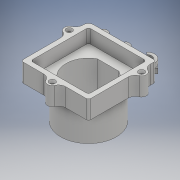
# Autodesk Inventor part: MS_FocusSliderv11
Saved by Autodesk Inventor 2017 (Build 210142000, 142)
## iProperties
Created: 2017-12-13
Part Number: MS_FocusSliderv11
Material: Generic
Document SubType Name: Modeling
Designer: andrew
Density: 1 g/cm^3
Appearance: Default
Author: andrew
Autodesk Inventor part; units mm, degrees
note: some values were not read from the file. Chosen so that the rebuilt part matches the saved one: edges of "Chamfer1".
ref_plane "YZ Plane" through (0, 0, 0) normal (1, 0, 0) x (0, 1, 0)
ref_plane "XZ Plane" through (0, 0, 0) normal (0, 1, 0) x (-1, 0, 0)
sketch "Sketch1" plane through (0, 0, 0) normal (0, 0, 1) x (1, 0, 0)
  circle A0 centre (0, 0) radius 5.75
  line L0 (2.2382, 4.0759) -> (-2.2382, 4.0759)
  arc A1 (-2.2382, 4.0759) -> (2.2382, 4.0759) centre (0, 0) ccw
  dimension "d0" = 11.5
  dimension "d50" = 9.3
  constraints: 2 centre point, 2 end point, 2 point on circle, 1 coincident
  measures "d0" diameter of A0
  measures "d50" diameter of A1
extrude "Extrusion1" add sketch "Sketch1" along normal blind 7
sketch "Sketch2" plane through (0, 0, 0) normal (0, 0, -1) x (-1, 0, 0)
  line L0 (-1.25, 5.125) -> (1.25, 5.125) construction
  circle A0 centre (0, 0) radius 5.75 construction
  line L1 (0, 0) -> (0, 9.5083) construction
  circle A1 centre (0, 0) radius 5.75 construction
  line L2 (0, 5.75) -> (0, 7.7304) construction
  line L3 (0, 5.125) -> (0, 7.5987) construction
  line L4 (-1.25, 5.125) -> (-1.25, 6.125) construction
  line L5 (-1.25, 6.125) -> (1.25, 6.125)
  line L6 (1.25, 6.125) -> (1.25, 4.5986)
  line L7 (1.25, 4.5986) -> (-1.25, 4.5986)
  line L8 (-1.25, 4.5986) -> (-1.25, 6.125)
  dimension "d3" = 2.5
  dimension "d4" = 1
  constraints: 18 end point, 3 vertical, 2 horizontal, 2 parallel, 2 point on line, 1 midpoint, 1 perpendicular, 1 vertical alignment, 1 other
  measures "d3" distance of L0.start L0.end
  measures "d4" distance of L0.start L4.end
extrude "Extrusion2" add sketch "Sketch2" against normal blind 5
sketch "Sketch3" plane through (0, 0, 7) normal (0, 0, 1) x (1, 0, 0)
  line L0 (6.5, 7) -> (-6, 7)
  arc A0 (-6, 7) -> (-7, 6) centre (-6, 6) ccw
  arc A1 (-7, -6.5) -> (-6.5, -7) centre (-6.5, -6.5) ccw
  arc A2 (6.5, -7) -> (7, -6.5) centre (6.5, -6.5) ccw
  arc A3 (7, 6.5) -> (6.5, 7) centre (6.5, 6.5) ccw
  line L1 (-5.5, 6) -> (5.5, 6)
  line L2 (6, 5.5) -> (6, -5.5)
  line L3 (5.5, -6) -> (-5.5, -6)
  line L4 (-6, -5.5) -> (-6, 5.5)
  arc A4 (-5.5, 6) -> (-6, 5.5) centre (-5.5, 5.5) ccw
  arc A5 (6, 5.5) -> (5.5, 6) centre (5.5, 5.5) ccw
  arc A6 (5.5, -6) -> (6, -5.5) centre (5.5, -5.5) ccw
  arc A7 (-6, -5.5) -> (-5.5, -6) centre (-5.5, -5.5) ccw
  line L5 (-10.9736, 8.9739) -> (-4.3472, 8.9739) construction
  arc A8 (-7.9, 4.4165) -> (-7.9, 2.5835) centre (-7.5, 3.5) ccw
  circle A9 centre (-7.5, 3.5) radius 0.375
  arc A10 (-0.9165, -7.9) -> (0.9165, -7.9) centre (0, -7.5) ccw
  circle A11 centre (0, -7.5) radius 0.375
  arc A12 (7.9, 2.5835) -> (7.9, 4.4165) centre (7.5, 3.5) ccw
  circle A13 centre (7.5, 3.5) radius 0.375
  line L6 (-7, 6) -> (-7, 5.7913)
  line L7 (-7, 1.2087) -> (-7, -6.5)
  arc A14 (-7.9, 4.4165) -> (-7, 5.7913) centre (-8.5, 5.7913) ccw
  arc A15 (-7, 1.2087) -> (-7.9, 2.5835) centre (-8.5, 1.2087) ccw
  line L8 (-6.5, -7) -> (-2.2913, -7)
  line L9 (2.2913, -7) -> (6.5, -7)
  arc A16 (-0.9165, -7.9) -> (-2.2913, -7) centre (-2.2913, -8.5) ccw
  arc A17 (2.2913, -7) -> (0.9165, -7.9) centre (2.2913, -8.5) ccw
  line L10 (7, -6.5) -> (7, 1.2087)
  line L11 (7, 5.7913) -> (7, 6.5)
  arc A18 (7, 5.7913) -> (7.9, 4.4165) centre (8.5, 5.7913) ccw
  arc A19 (7.9, 2.5835) -> (7, 1.2087) centre (8.5, 1.2087) ccw
  arc A20 (-2.2382, 4.0759) -> (2.2382, 4.0759) centre (0, 0) ccw
  line L12 (-2.2382, 4.0759) -> (2.2382, 4.0759) projected
  line L13 (2.2382, 4.0759) -> (-2.3054, 4.0383)
  arc A21 (2.2382, -4.0759) -> (2.2382, 4.0759) centre (0, 0) ccw
  arc A22 (-2.2382, 4.0759) -> (-2.2382, -4.0759) centre (0, 0) ccw
  point P0 (7, -7)
  point P1 (-7, -7)
  point P2 (7, 7)
  point P3 (-7, 4.366)
  point P4 (-7, 2.634)
  point P5 (-0.866, -7)
  point P6 (0.866, -7)
  point P7 (7, 2.634)
  point P8 (7, 4.366)
  constraints: 48 point on circle, 27 end point, 23 centre point, 7 coincident, 7 point on line
extrude "Extrusion3" add sketch "Sketch3" along normal blind 1 contours A3 L11 A18 A12 A19 L10 A2 L9 A17 A10 A16 L8 A1 L7 A15 A8 A14 L6 A0 L0 | L1 A5 L2 A6 L3 A7 L4 A4
sketch "Sketch4" plane through (0, 0, 8) normal (0, 0, 1) x (1, 0, 0)
  arc A0 (-5.5, 6) -> (-6, 5.5) centre (-5.5, 5.5) ccw
  line L0 (-5.5, 6) -> (5.5, 6)
  line L1 (-6, -5.5) -> (-6, 5.5)
  line L2 (-7, 1.2087) -> (-7, -6.5)
  arc A1 (-6, -5.5) -> (-5.5, -6) centre (-5.5, -5.5) ccw
  line L3 (6.5, 7) -> (-6, 7)
  line L4 (6, 5.5) -> (6, -5.5)
  line L5 (7, -6.5) -> (7, 1.2087)
  line L6 (5.5, -6) -> (-5.5, -6)
  arc A2 (5.5, -6) -> (6, -5.5) centre (5.5, -5.5) ccw
  circle A3 centre (7.5, 3.5) radius 0.375
  arc A4 (7.9, 2.5835) -> (7, 1.2087) centre (8.5, 1.2087) ccw
  arc A5 (7, 5.7913) -> (7.9, 4.4165) centre (8.5, 5.7913) ccw
  arc A6 (7.9, 2.5835) -> (7.9, 4.4165) centre (7.5, 3.5) ccw
  arc A7 (6, 5.5) -> (5.5, 6) centre (5.5, 5.5) ccw
  line L7 (7, 5.7913) -> (7, 6.5)
  arc A8 (7, 6.5) -> (6.5, 7) centre (6.5, 6.5) ccw
  arc A9 (-6, 7) -> (-7, 6) centre (-6, 6) ccw
  line L8 (-10.9736, 8.9739) -> (-4.3472, 8.9739) construction
  arc A10 (-7.9, 4.4165) -> (-7.9, 2.5835) centre (-7.5, 3.5) ccw
  circle A11 centre (-7.5, 3.5) radius 0.375
  arc A12 (-7, 1.2087) -> (-7.9, 2.5835) centre (-8.5, 1.2087) ccw
  line L9 (-7, 6) -> (-7, 5.7913)
  arc A13 (-7.9, 4.4165) -> (-7, 5.7913) centre (-8.5, 5.7913) ccw
  arc A14 (-7, -6.5) -> (-6.5, -7) centre (-6.5, -6.5) ccw
  arc A15 (6.5, -7) -> (7, -6.5) centre (6.5, -6.5) ccw
  arc A16 (-0.9165, -7.9) -> (0.9165, -7.9) centre (0, -7.5) ccw
  circle A17 centre (0, -7.5) radius 0.375
  line L10 (2.2913, -7) -> (6.5, -7)
  arc A18 (-0.9165, -7.9) -> (-2.2913, -7) centre (-2.2913, -8.5) ccw
  arc A19 (2.2913, -7) -> (0.9165, -7.9) centre (2.2913, -8.5) ccw
  line L11 (-6.5, -7) -> (-2.2913, -7)
  arc A20 (-2.2382, 4.0759) -> (2.2382, 4.0759) centre (0, 0) ccw
  line L12 (-2.2382, 4.0759) -> (2.2382, 4.0759)
  line L13 (2.2382, 4.0759) -> (-2.3054, 4.0383)
  arc A21 (2.2382, -4.0759) -> (2.2382, 4.0759) centre (0, 0) ccw
  arc A22 (-2.2382, 4.0759) -> (-2.2382, -4.0759) centre (0, 0) ccw
  point P0 (7, 4.366)
  point P1 (7, 2.634)
  point P2 (7, 7)
  point P3 (-7, 2.634)
  point P4 (-7, 4.366)
  point P5 (7, -7)
  point P6 (-7, -7)
  point P7 (-0.866, -7)
  point P8 (0.866, -7)
  constraints: 48 point on circle, 29 end point, 23 centre point, 7 coincident, 7 point on line
extrude "Extrusion4" add sketch "Sketch4" along normal blind 2.8 contours A12 A10 A13 L9 A9 L3 A8 L7 A5 A6 A4 L5 A15 L10 A19 A16 A18 L11 A14 L2
sketch "Sketch5" plane through (-1.25, 6.125, 0) normal (0, 1, 0) x (1, 0, 0)
  line L0 (1.8283, -3.8925) -> (1.8437, -3.7979)
  line L1 (0.8374, -4.1796) -> (0.9116, -4.2402)
  line L2 (0.7226, -3.4732) -> (0.7738, -3.3922)
  line L3 (1.7534, -0.9317) -> (1.798, -1.0165)
  line L4 (0.8374, -1.6796) -> (0.9116, -1.7402)
  line L5 (0.7738, -0.8922) -> (0.8374, -0.8204)
  line L6 (0, 0) -> (2.5, 0)
  line L7 (0, 0) -> (0, -5)
  circle A0 centre (1.25, -1.25) radius 0.5937
  circle A1 centre (1.25, -3.75) radius 0.5937
  point P0 (1.25, 0)
  point P1 (1.0843, -1.8221)
  dimension "d40" = 1.1874
  constraints: 16 end point, 6 tangent, 2 centre point
  measures "d40" diameter of A1
extrude "Extrusion5" cut sketch "Sketch5" against normal blind 5
fillet "Fillet1" radius 2 2 edges at (-1.25, 5.6125, 2.5) (1.25, 5.6125, 2.5)
chamfer "Chamfer1" distance 0.5 angle 45 1 edges at (0, 4.0759, 0)
sketch "Sketch6" plane through (0, 0, 7) normal (0, 0, -1) x (-1, 0, 0)
  arc A0 (0, 7.125) -> (-0.2652, 7.7652) centre (0, 7.5) ccw
  arc A1 (0.9165, 7.9) -> (-0.7071, 8.2071) centre (0, 7.5) ccw
  arc A2 (0.9165, 7.9) -> (1.6918, 7.125) centre (2.2913, 8.5) ccw
  line L0 (0, 7.125) -> (-1.6918, 7.125)
  arc A3 (-3.7231, 7) -> (-5.2965, 8.2067) centre (-4.5894, 7.4996) ccw
  line L1 (4.5826, 7) -> (4.5826, 6.4945)
  arc A4 (4.5826, 7.125) -> (4.2559, 7.6842) centre (4.5826, 7.5) ccw
  arc A5 (5.4991, 7.9) -> (3.5997, 7.6842) centre (4.5826, 7.5) ccw
  line L2 (2.2913, 7) -> (6, 7)
  arc A6 (5.4991, 7.9) -> (5.569, 7.7602) centre (6.8739, 8.5) ccw
  line L3 (4.5826, 7.125) -> (1.6918, 7.125)
  line L4 (4.2559, 7.6842) -> (3.5997, 7.6842)
  line L5 (6, 7) -> (5.569, 7.7602)
  arc A7 (-6.5, 7) -> (-7, 6.5) centre (-6.5, 6.5) ccw projected
  arc A8 (-3.1, 8.1496) -> (-1.6918, 7.125) centre (-1.4159, 8.9843) ccw
  arc A9 (-3.1, 8.1496) -> (-5.7384, 8.6487) centre (-4.5894, 7.4996) ccw
  line L6 (-5.2965, 8.2067) -> (-5.7384, 8.6487)
  line L7 (-4.5894, 7.4996) -> (-2.9644, 7.4996) construction
  line L8 (-0.2652, 7.7652) -> (-0.7071, 8.2071)
  line L9 (0, 7.5) -> (1, 7.5) construction
  line L10 (-3.7231, 7) -> (2.2913, 7)
  line L11 (6, 7) -> (-6.5, 7) projected
  point P0 (0, 0)
  point P1 (-6.5196, 6.9996)
  point P2 (2.8908, 7.125)
  dimension "d57" = 135
  dimension "d58" = 135
  constraints: 22 end point, 20 point on circle, 9 centre point, 3 point on line, 2 horizontal, 1 coincident, 1 tangent
  measures "d57" angle of L7 L6
  measures "d58" angle of L9 L8
extrude "Extrusion6" add sketch "Sketch6" against normal blind 1
ref_plane "Work Plane1" through (0, 0, 8.75) normal (0, 0, 1) x (1, 0, 0)
sketch "Sketch7" plane through (0, 0, 8.75) normal (0, 0, 1) x (1, 0, 0)
  line L0 (-4.5894, 7.4996) -> (-2.9644, 7.4996) construction
  line L1 (0, 7.5) -> (1, 7.5) construction
  arc A0 (0, 10.0353) -> (-0.2652, 10.6754) centre (0, 10.4103) ccw
  arc A1 (0.9165, 10.8103) -> (-0.7071, 11.1174) centre (0, 10.4103) ccw
  arc A2 (0.9165, 10.8103) -> (2.2913, 9.9103) centre (2.2913, 11.4103) ccw
  line L2 (0, 10.0353) -> (-1.6918, 10.0353)
  arc A3 (-3.7231, 9.9103) -> (-5.2965, 11.117) centre (-4.5894, 10.4099) ccw
  line L3 (4.5826, 9.9103) -> (4.5826, 9.4048)
  arc A4 (4.5826, 10.0353) -> (4.2559, 10.5944) centre (4.5826, 10.4103) ccw
  arc A5 (5.4991, 10.8103) -> (3.5997, 10.5944) centre (4.5826, 10.4103) ccw
  line L4 (2.2913, 9.9103) -> (6, 9.9103)
  arc A6 (5.4991, 10.8103) -> (5.569, 10.6704) centre (6.8739, 11.4103) ccw
  line L5 (4.5826, 10.0353) -> (2.8908, 10.0353)
  line L6 (4.2559, 10.5944) -> (3.5997, 10.5944)
  arc A7 (2.2913, 9.9103) -> (2.8908, 10.0353) centre (2.2913, 11.4103) ccw
  line L7 (6, 9.9103) -> (5.569, 10.6704)
  arc A8 (-6.5, 9.9103) -> (-7, 9.4103) centre (-6.5, 9.4103) ccw
  arc A9 (-3.1, 11.0599) -> (-1.6918, 10.0353) centre (-1.4159, 11.8945) ccw
  arc A10 (-3.1, 11.0599) -> (-5.7384, 11.5589) centre (-4.5894, 10.4099) ccw
  line L8 (-5.2965, 11.117) -> (-5.7384, 11.5589)
  line L9 (-4.5894, 10.4099) -> (-2.9644, 10.4099) construction
  line L10 (-0.2652, 10.6754) -> (-0.7071, 11.1174)
  line L11 (0, 10.4103) -> (1, 10.4103) construction
  line L12 (-3.7231, 9.9103) -> (2.2913, 9.9103)
  line L13 (6, 9.9103) -> (-6.5, 9.9103)
  line L14 (-4.5894, 10.4099) -> (-6.5589, 10.5944)
  line L15 (0, 10.4103) -> (-1.6918, 10.8103)
  line L16 (4.5826, 10.4103) -> (2.0631, 10.4103)
  arc A11 (5.4486, 7) -> (3.8755, 8.2071) centre (4.5826, 7.5) ccw
  line L17 (3.8755, 8.2071) -> (3.4335, 8.649)
  arc A12 (6.2076, 7.5) -> (3.4335, 8.649) centre (4.5826, 7.5) ccw
  arc A13 (6.2076, 7.5) -> (6.5, 7) centre (6.894, 7.5659) ccw
  arc A14 (0, 7.125) -> (-0.2652, 7.7652) centre (0, 7.5) ccw
  arc A15 (0.9165, 7.9) -> (-0.7071, 8.2071) centre (0, 7.5) ccw
  line L18 (-0.2652, 7.7652) -> (-0.7071, 8.2071)
  line L19 (6.5, 7) -> (-6, 7)
  line L20 (-3.7231, 7) -> (2.2913, 7)
  line L21 (0, 7.5) -> (1, 7.5) construction
  arc A16 (0.9165, 7.9) -> (2.2913, 7) centre (2.2913, 8.5) ccw
  line L22 (0, 7.125) -> (-3.243, 7.125)
  line L23 (2.2913, 7) -> (6, 7)
  line L24 (-4.5894, 6.9996) -> (-4.5894, 6.4941)
  arc A17 (-4.5894, 7.1246) -> (-4.916, 7.6838) centre (-4.5894, 7.4996) ccw
  arc A18 (-3.6728, 7.8996) -> (-5.5722, 7.6838) centre (-4.5894, 7.4996) ccw
  line L25 (-4.5894, 6.9996) -> (-3.1719, 6.9996)
  arc A19 (-6.8806, 6.9996) -> (-6.8468, 7) centre (-6.8806, 8.4996) ccw
  line L26 (-4.916, 7.6838) -> (-5.5722, 7.6838)
  line L27 (-4.5894, 7.1246) -> (-5.9293, 7.1246)
  arc A20 (-3.6728, 7.8996) -> (-3.6029, 7.7598) centre (-2.2981, 8.4996) ccw
  line L28 (-5.569, 7.7602) -> (-6, 7) projected
  line L29 (-5.9293, 7.1246) -> (-6, 7)
  line L30 (-3.1719, 6.9996) -> (-4.5894, 6.9996)
  line L31 (-3.1719, 6.9996) -> (-3.1721, 7)
  line L32 (-3.243, 7.125) -> (-3.6029, 7.7598)
  point P0 (0, 0)
  point P1 (-6.5196, 9.9099)
  dimension "d61" = 135
  dimension "d62" = 135
  dimension "d64" = 135
  constraints: 64 end point, 46 point on circle, 21 centre point, 8 point on line, 6 horizontal, 3 tangent, 2 coincident, 1 collinear
  measures "d61" angle of L9 L8
  measures "d62" angle of L11 L10
  measures "d64" angle of L21 L18
extrude "Extrusion7" add sketch "Sketch7" along normal blind 1 contours A11 L17 A12 A13 L19 | A14 L18 A15 A16 L19 L28 L27 A17 L26 A18 A20 L32 L22
chamfer "Chamfer2" distance 0.25 distance2 0.5 1 edges at (-0.375, -7.5, 10.8) measured on face at (2, 6.6667, 10.8)
chamfer "Chamfer3" distance 0.25 distance2 0.5 1 edges at (7.125, 3.5, 10.8) measured on face at (2, 6.6667, 10.8)
chamfer "Chamfer4" distance 0.25 distance2 0.5 1 edges at (-7.875, 3.5, 10.8) measured on face at (2, 6.6667, 10.8)
body "Solid1"
